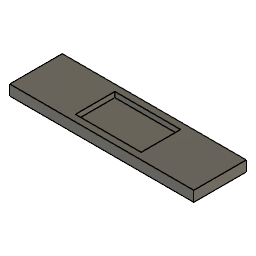
Canal - middle plate v1 (Autodesk Fusion 360 design; units mm, degrees)
Autodesk Fusion 360 part; units mm, degrees
sketch "Esquisse1" plane through (0, 0, 0) normal (0, 0, 1) x (1, 0, 0)
  line L0 (0, 40) -> (70, 40)
  line L1 (70, 40) -> (70, 20)
  line L2 (70, 20) -> (0, 20)
  line L3 (0, 20) -> (0, 40)
  dimension "d1" = 70
  dimension "d2" = 20
  constraint horizontal L0
  constraint vertical L1
  constraint horizontal L2
  constraint vertical L3
  measures "d1" distance of L1 L3
  measures "d2" distance of L0 L2
extrude "Extrusion1" add sketch "Esquisse1" along normal blind 4
sketch "Esquisse2" plane through (0, 0, 0) normal (0, 0, -1) x (1, 0, 0)
  line L0 (70, -20) -> (0, -20)
  line L1 (0, -20) -> (0, -40)
  line L2 (0, -40) -> (70, -40)
  line L3 (70, -40) -> (70, -20)
  line L4 (7.5, -23) -> (12.5, -23)
  line L5 (12.5, -23) -> (12.5, -25)
  line L6 (12.5, -25) -> (7.5, -25)
  line L7 (7.5, -25) -> (7.5, -23)
  line L8 (10, -23) -> (10, -25) construction
  line L9 (35, -20) -> (35, -40) construction
  line L10 (57.5, -23) -> (57.5, -25)
  line L11 (62.5, -23) -> (57.5, -23)
  line L12 (62.5, -25) -> (62.5, -23)
  line L13 (57.5, -25) -> (62.5, -25)
  line L14 (0, -30) -> (70, -30) construction
  line L15 (7.5, -37) -> (12.5, -37)
  line L16 (12.5, -37) -> (12.5, -35)
  line L17 (12.5, -35) -> (7.5, -35)
  line L18 (7.5, -35) -> (7.5, -37)
  line L19 (62.5, -37) -> (57.5, -37)
  line L20 (62.5, -35) -> (62.5, -37)
  line L21 (57.5, -35) -> (62.5, -35)
  line L22 (57.5, -37) -> (57.5, -35)
  dimension "d5" = 25
  constraint horizontal L4
  constraint vertical L5
  constraint horizontal L6
  constraint vertical L7
  constraint midpoint L4 L8.start
  constraint midpoint L6 L8.end
  constraint midpoint L0 L9.start
  constraint midpoint L2 L9.end
  constraint symmetric L4.start L9 L11.start
  constraint symmetric L4.end L9 L10.start
  constraint symmetric L5.end L9 L10.end
  constraint symmetric L6.end L9 L12.start
  constraint midpoint L1 L14.start
  constraint midpoint L3 L14.end
  constraint symmetric L4.start L14 L15.start
  constraint symmetric L4.end L14 L15.end
  constraint symmetric L5.end L14 L16.end
  constraint symmetric L6.end L14 L17.end
  constraint symmetric L10.start L14 L19.end
  constraint symmetric L10.end L14 L21.start
  constraint symmetric L11.start L14 L19.start
  constraint symmetric L12.start L14 L20.start
  measures "d5" distance of L8 L9
extrude "Extrusion2" cut sketch "Esquisse2" against normal blind 2 contours L4 L5 L6 L7 | L10 L11 L12 L13 | L15 L16 L17 L18 | L19 L20 L21 L22
sketch "Esquisse3" plane through (0, 0, 4) normal (0, 0, 1) x (-1, 0, 0)
  line L0 (0, -20) -> (-70, -20)
  line L1 (-70, -20) -> (-70, -40)
  line L2 (-70, -40) -> (0, -40)
  line L3 (0, -40) -> (0, -20)
  line L4 (-22.5, -37.5) -> (-47.5, -37.5)
  line L5 (-47.5, -37.5) -> (-47.5, -22.5)
  line L6 (-47.5, -22.5) -> (-22.5, -22.5)
  line L7 (-22.5, -22.5) -> (-22.5, -37.5)
  line L8 (0, -30) -> (-70, -30) construction
  line L9 (-35, -40) -> (-35, -20) construction
  dimension "d8" = 25
  dimension "d9" = 15
  constraint horizontal L4
  constraint vertical L5
  constraint horizontal L6
  constraint vertical L7
  constraint midpoint L3 L8.start
  constraint midpoint L1 L8.end
  constraint midpoint L2 L9.start
  constraint midpoint L0 L9.end
  constraint symmetric L5 L7 L9
  constraint symmetric L0 L2 L8
  constraint symmetric L4 L6 L8
  measures "d8" distance of L5 L7
  measures "d9" distance of L4 L6
extrude "Extrusion3" cut sketch "Esquisse3" against normal blind 2 contours L4 L5 L6 L7
